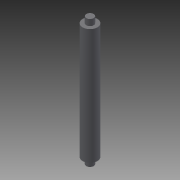
# Autodesk Inventor part: 022.08-FO1_BM_r
Saved by Autodesk Inventor 2014 (Build 180170000, 170)
## iProperties
Created: 2014-01-19
Part Number: 022.08-FO1_BM_r
Material: Generic
Catalog Web Link: www.cadenas.de
Description: FO1_basic_model_r-Bimba FLAT-1
Vendor: BIMBA
Document SubType Name: Standard Catalog Part
Designer: Andrew Toennies
Manufacturer: BIMBA
Density: 1 g/cm^3
Appearance: RGB(180.00000447034725,180.00000447034725,180.00000447034725)
Category: PARTsolutions
Company: BIMBA
Title: 022.08-FO1_BM_r
Author: Cadenas PARTsolutions
Comments: Bimba FLAT-1
PSOL_IDENT_0: {$CADENAS_DATA\23d-libs\bimba\bimba\bimba_imperial\bimba_full_line\flat_cylinders\fo1\fo1_basic_mode
PSOL_IDENT_1: l_r.prj},189 {VTYP=3D},{NB=022.08-FO1_BM_r},{LINA=022.08-FO1_BM_r},{NN=FO1_basic_model_r},{DATE=28.0
PSOL_IDENT_2: 9.2011 06:27:30},{GEOMDATE=28.09.2011 05:59:00},{VERSION=},{LINEID=10},{LINESUBID=-1},{WBVAR=STROKE}
PSOL_IDENT_3: {NB=022.08-FO1_BM_r},{LINA=022.08-FO1_BM_r},{KT=DUMMY},{PN=022.08-FO1_BM_r},{BORE=0.56250000},{BOR
PSOL_IDENT_4: EPN=02},{STROKE=2.08},{CPIL=0.11800000},{RD=0.24000},{RD1=0.12000000},{CH=0.03000000},{TDDP=0.100000
PSOL_IDENT_5: 00},{STROKEMIN=0.202}
CNS_NN: FO1_basic_model_r
CNS_NT: Bimba FLAT-1
CNS_NB: 022.08-FO1_BM_r
CNS_NBSYN: $PN.
CNS_LINA: 022.08-FO1_BM_r
CNS_PN: 022.08-FO1_BM_r
CNS_BORE: 9/16
CNS_BOREPN: 02
CNS_STROKE: 2.080
CNS_CPIL: 0.11800000
CNS_RD: 0.24000
CNS_RD1: 0.12000000
CNS_CH: 0.03000000
CNS_TDDP: 0.10000000
CNS_STROKEMIN: 0.202
SUPPLIER: BIMBA
ARTICLENO: 022.08-FO1_BM_r
BOMINFO: 022.08-FO1_BM_r
CREATOR: CADENAS GmbH
Autodesk Inventor part; units mm, degrees
ref_plane "YZ Plane" through (0, 0, 0) normal (1, 0, 0) x (0, 1, 0)
ref_plane "XZ Plane" through (0, 0, 0) normal (0, 1, 0) x (-1, 0, 0)
ref_plane "XY Plane" through (0, 0, 0) normal (0, 0, 1) x (1, 0, 0)
sketch "Sketch_1" plane through (0, 0, 0) normal (0, 0, 1) x (1, 0, 0)
  line L0 (0, 0) -> (0, 52.832)
  line L1 (0, 52.832) -> (3.048, 52.832)
  line L2 (3.048, 52.832) -> (3.048, 0)
  line L3 (3.048, 0) -> (0, 0)
  line L4 (0, 0) -> (0, 52.832)
  constraints: 10 end point
revolve "Revolution1" add sketch "Sketch_1" angle 360 about axis through (0, 0, 0) along (0, -1, 0)
sketch "Sketch_3" plane through (0, 0, 0) normal (0, 0, 1) x (1, 0, 0)
  line L0 (0, 0) -> (0, 2.54)
  line L1 (1.524, 0) -> (3.048, 0)
  line L2 (3.048, 0) -> (3.048, 2.54)
  line L3 (3.048, 2.54) -> (1.524, 2.54)
  line L4 (1.524, 2.54) -> (1.524, 0)
  constraints: 10 end point
revolve "Revolution2" cut sketch "Sketch_3" angle 360 about axis through (0, 0, 0) along (0, -1, 0)
sketch "Sketch_4" plane through (0, 0, 0) normal (0, 0, 1) x (1, 0, 0)
  line L0 (0, 50.292) -> (0, 52.832)
  line L1 (1.524, 52.832) -> (1.524, 50.292)
  line L2 (1.524, 50.292) -> (3.048, 50.292)
  line L3 (3.048, 50.292) -> (3.048, 52.832)
  line L4 (3.048, 52.832) -> (1.524, 52.832)
  constraints: 10 end point
revolve "Revolution3" cut sketch "Sketch_4" angle 360 about axis through (0, 50.292, 0) along (0, -1, 0)
ref_plane "additional_rod_XY" through (0, 0, 0) normal (0, 1, 0) x (1, 0, 0)
ref_plane "additional_rod_YZ" through (0, 0, 0) normal (1, 0, 0) x (0, 0, -1)
ref_plane "additional_rod_ZX" through (0, 0, 0) normal (0, 0, -1) x (0, 1, 0)
body "Solid1"
